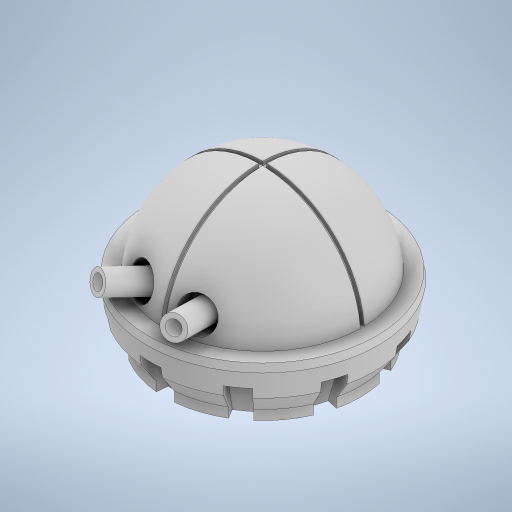
# Autodesk Inventor part: 屋頂-3
Saved by Autodesk Inventor 2024 (Build 280153000, 153)
## iProperties
Created: 2024-05-18
Part Number: 屋頂-3
Material: 一般
Document SubType Name: Modeling
Designer: User
Density: 1 g/cm^3
Appearance: 預設
Author: User
Autodesk Inventor part; units mm, degrees
ref_plane "YZ Plane" through (0, 0, 0) normal (1, 0, 0) x (0, 1, 0)
ref_plane "XZ Plane" through (0, 0, 0) normal (0, 1, 0) x (-1, 0, 0)
ref_plane "XY Plane" through (0, 0, 0) normal (0, 0, 1) x (1, 0, 0)
sketch "草圖1" plane through (0, 0, 0) normal (0, 1, 0) x (-1, 0, 0)
  circle A0 centre (0, 0) radius 26
  circle A1 centre (0, 0) radius 30
  line L0 (0, 26) -> (0, -26)
  dimension "d0" = 52
  dimension "d1" = 60
  constraints: 2 centre point, 2 coincident, 2 end point, 2 point on circle, 1 vertical
  measures "d0" diameter of A0
  measures "d1" diameter of A1
revolve "迴轉1" add sketch "草圖1" angle 180 about axis through (0, 0, 26) along (0, 0, 1) picked at (-10.6775, 1.2965) contours L0 A0
sketch "草圖2" plane through (0, 0, 0) normal (0, -1, 0) x (1, 0, 0)
  circle A0 centre (0, 0) radius 30
  dimension "d3" = 60
  constraints: 1 centre point, 1 coincident
  measures "d3" diameter of A0
extrude "擠出1" add sketch "草圖2" along normal blind 6.5 draft -10 and the other way blind 2 draft -10
sketch "草圖3" plane through (0, 0, 0) normal (1, 0, 0) x (0, 1, 0)
  line L0 (2, -25.923) -> (2, 25.923) projected
  arc A0 (2, -25.923) -> (2, 25.923) centre (0, 0) ccw
  arc A1 (2, -25.923) -> (2, 25.923) centre (0, 0) ccw projected
  line L1 (2, 25.923) -> (2, -25.923)
  arc A2 (2, -24.9199) -> (2, 24.9199) centre (0, 0) ccw
  point P0 (2, 24.9199)
  point P1 (2, -24.9199)
  dimension "d8" = 1
  constraints: 4 point on circle, 2 centre point, 2 concentric, 2 end point, 2 point on line, 1 collinear
  measures "d8" radial gap between concentric circles of A0 A2
extrude "擠出2" cut sketch "草圖3" along normal mid plane 1 contours L0 A2 A0
sketch "草圖4" plane through (0, 0, 0) normal (0, 0, 1) x (1, 0, 0)
  line L0 (25.923, 2) -> (0.5, 2) projected
  line L1 (-0.5, 2) -> (-25.923, 2) projected
  line L2 (-0.5, 25.9952) -> (-0.5, 2) projected
  arc A0 (25.923, 2) -> (-25.923, 2) centre (0, 0) ccw
  line L3 (25.923, 2) -> (-25.923, 2)
  arc A1 (24.9199, 2) -> (-24.9199, 2) centre (0, 0) ccw
  point P0 (0, 0)
  point P1 (-24.9199, 2)
  point P2 (24.9199, 2)
  dimension "d11" = 1
  constraints: 5 point on circle, 2 centre point, 2 end point, 2 point on line, 1 collinear, 1 concentric
  measures "d11" radial gap between concentric circles of A0 A1
extrude "擠出3" cut sketch "草圖4" along normal mid plane 1 contours L0 A1 L2 A0 | L2 A1 L1 A0
ref_plane "工作平面1" through (0, 0, 0) normal (-0.315329, 0.2747861, 0.9083283) x (-0.6569774, -0.7539102, 0)
ref_plane "工作平面2" through (0, 0, 0) normal (0.2638739, 0.2792959, 0.9232358) x (-0.7268903, 0.6867535, 0)
sketch "草圖6" plane through (0, 0, 0) normal (-0.315329, 0.2747861, 0.9083283) x (-0.6569774, -0.7539102, 0)
  circle A0 centre (0, 0) radius 1.8
  circle A1 centre (0, 0) radius 2.9
  dimension "d20" = 3.6
  dimension "d21" = 5.8
  constraints: 2 centre point, 2 coincident
  measures "d20" diameter of A0
  measures "d21" diameter of A1
extrude "擠出5" add sketch "草圖6" along normal blind 35 contours A0 | A1
sketch "草圖7" plane through (-11.0365, 9.6175, 31.7915) normal (-0.315329, 0.2747861, 0.9083283) x (0.9446939, 0, 0.3279534)
  circle A0 centre (0, 0) radius 2.9
  circle A1 centre (0, 0) radius 1.8
  circle A2 centre (0, 0) radius 4.4
  point P0 (0, 0)
  dimension "d24" = 5.8
  dimension "d25" = 3.6
  dimension "d26" = 8.8
  constraints: 3 centre point, 3 coincident
  measures "d24" diameter of A0
  measures "d25" diameter of A1
  measures "d26" diameter of A2
extrude "擠出6" cut sketch "草圖7" against normal blind 10 contours A1
extrude "擠出7" cut sketch "草圖7" against normal blind 15 contours A2
sketch "草圖8" plane through (0, 0, 0) normal (0.2638739, 0.2792959, 0.9232358) x (-0.7268903, 0.6867535, 0)
  circle A0 centre (0, 0) radius 2.95
  dimension "d31" = 5.9
  constraints: 1 centre point, 1 coincident
  measures "d31" diameter of A0
extrude "擠出8" add sketch "草圖8" along normal blind 35
sketch "草圖9" plane through (9.2356, 9.7754, 32.3133) normal (0.2638739, 0.2792959, 0.9232358) x (0.9614986, 0, -0.27481)
  circle A0 centre (0, 0) radius 2.95
  circle A1 centre (0, 0) radius 1.75
  circle A2 centre (0, 0) radius 4.3
  dimension "d34" = 5.9
  dimension "d35" = 3.5
  dimension "d36" = 8.6
  constraints: 3 centre point, 3 coincident
  measures "d34" diameter of A0
  measures "d35" diameter of A1
  measures "d36" diameter of A2
extrude "擠出9" cut sketch "草圖9" against normal blind 10 contours A1
extrude "擠出10" cut sketch "草圖9" against normal blind 15 contours A2
sketch "草圖10" plane through (0, -6.5, 0) normal (0, -1, 0) x (1, 0, 0)
  line L0 (-0.5, -0.5) -> (0, 0) projected
  circle A0 centre (0, 0) radius 28.8539
  constraints: 1 centre point, 1 coincident
extrude "擠出11" add sketch "草圖10" along normal blind 5 draft -35
sketch "草圖11" plane through (0, -11.5, 0) normal (0, -1, 0) x (1, 0, 0)
  circle A0 centre (0, 0) radius 25.3528
  constraints: 1 centre point, 1 coincident
extrude "擠出12" add sketch "草圖11" along normal blind 2.5
sketch "草圖12" plane through (0, -14, 0) normal (0, -1, 0) x (1, 0, 0)
  circle A0 centre (0, 0) radius 30
  line L0 (0, 0) -> (0, -30)
  circle A1 centre (0, 0) radius 30 projected
  line L1 (0, 0) -> (-2.8, -29.869)
  line L2 (0, 0) -> (-0.5, 0.5) projected
  line L3 (2.8, -29.869) -> (0, 0)
  line L4 (19.8218, -22.5188) -> (0, 0)
  line L5 (0, 0) -> (15.2913, -25.8104)
  line L6 (29.2724, -6.5671) -> (0, 0)
  line L7 (0, 0) -> (27.5419, -11.893)
  line L8 (27.5419, 11.893) -> (0, 0)
  line L9 (0, 0) -> (29.2724, 6.5671)
  line L10 (15.2913, 25.8104) -> (0, 0)
  line L11 (0, 0) -> (19.8218, 22.5188)
  line L12 (-2.8, 29.869) -> (0, 0)
  line L13 (0, 0) -> (2.8, 29.869)
  line L14 (-19.8218, 22.5188) -> (0, 0)
  line L15 (0, 0) -> (-15.2913, 25.8104)
  line L16 (-29.2724, 6.5671) -> (0, 0)
  line L17 (0, 0) -> (-27.5419, 11.893)
  line L18 (-27.5419, -11.893) -> (0, 0)
  line L19 (0, 0) -> (-29.2724, -6.5671)
  line L20 (-15.2913, -25.8104) -> (0, 0)
  line L21 (0, 0) -> (-19.8218, -22.5188)
  circle A2 centre (0, 0) radius 22.5
  point P0 (-21.9543, 4.9253)
  point P1 (-20.6564, 8.9198)
  point P2 (-20.6564, -8.9198)
  point P3 (-21.9543, -4.9253)
  point P4 (-11.4685, -19.3578)
  point P5 (-14.8664, -16.8891)
  point P6 (2.1, -22.4018)
  point P7 (-2.1, -22.4018)
  point P8 (14.8664, -16.8891)
  point P9 (11.4685, -19.3578)
  point P10 (21.9543, -4.9253)
  point P11 (20.6564, -8.9198)
  point P12 (20.6564, 8.9198)
  point P13 (21.9543, 4.9253)
  point P14 (11.4685, 19.3578)
  point P15 (14.8664, 16.8891)
  point P16 (-2.1, 22.4018)
  point P17 (2.1, 22.4018)
  point P18 (-14.8664, 16.8891)
  point P19 (-11.4685, 19.3578)
  dimension "d48" = 60
  dimension "d47" = 5.6
  dimension "d49" = 2.8
  dimension "d52" = 360
  dimension "d54" = 45
  constraints: 42 end point, 4 coincident, 2 point on circle, 2 vertical, 1 centre point, 62 other
  measures "d47" distance of L1.end L3.start
  measures "d49" distance from line of L0 L1.end
  measures "d54" diameter of A2
extrude "擠出13" cut sketch "草圖12" against normal blind 10 contours L9 A2 L8 A0 | A0 L7 A2 L6 | L11 A2 L10 A0 | A0 L5 A2 L4 | A2 L3 A0 L0 | L0 A0 L1 A2 | L12 A0 L13 A2 | L14 A0 L15 A2 | L16 A0 L17 A2 | L18 A0 L19 A2 | L20 A0 L21 A2
draft "面拔模1" angle 20 pull direction (0, -1, 0) fixed plane through (-6.069, -14, 2.9172) normal (0, -1, 0) faces at (-21.8473, -10.6667, 5.3802) (-11.8681, -7.3333, 19.1154) (1.6343, -7.3333, 22.4406) (13.4135, -7.3333, 18.0646) (20.8372, -10.6667, 8.4888) (20.8372, -7.3333, -8.4888) (11.8681, -7.3333, -19.1154) (-1.1678, -7.3333, -22.4697) (-14.5124, -7.3333, -17.1942) (-21.7308, -7.3333, -5.8328)
